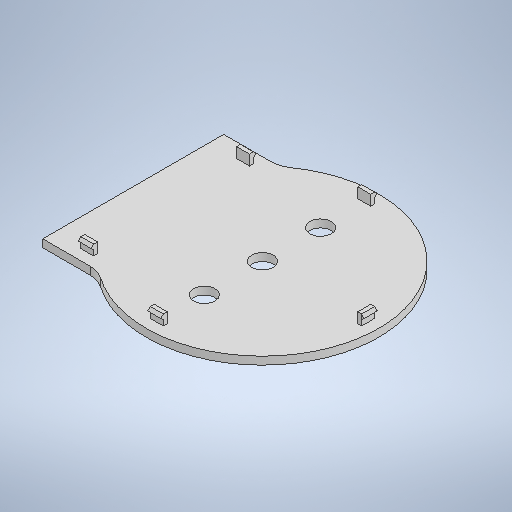
# Autodesk Inventor part: SCARA arm base - lid
Saved by Autodesk Inventor 2025.2 (Build 292293000, 293)
## iProperties
Created: 2025-01-29
Part Number: SCARA arm base - lid
Material: Generic
Document SubType Name: Modeling
Designer: caomi
Density: 1 g/cm^3
Appearance: Default
Author: caomi
Autodesk Inventor part; units mm, degrees
ref_plane "YZ Plane" through (0, 0, 0) normal (1, 0, 0) x (0, 1, 0)
ref_plane "XZ Plane" through (0, 0, 0) normal (0, 1, 0) x (-1, 0, 0)
ref_plane "XY Plane" through (0, 0, 0) normal (0, 0, 1) x (1, 0, 0)
sketch "Sketch1" plane through (0, 0, 0) normal (0, 1, 0) x (-1, 0, 0)
  circle A0 centre (0, 0) radius 45
  line L0 (28.2843, 35) -> (50, 35)
  line L1 (50, 35) -> (50, -35)
  line L2 (50, -35) -> (28.2843, -35)
  dimension "d0" = 90
  dimension "d1" = 70
  dimension "d2" = 50
  constraints: 6 end point, 2 perpendicular, 2 point on circle, 1 centre point, 1 coincident, 1 horizontal, 1 vertical alignment
  measures "d0" diameter of A0
  measures "d1" distance of L0.end L1.end
  measures "d2" distance from line of point (0, 0) L1
extrude "Extrusion1" add sketch "Sketch1" along normal blind 3
fillet "Fillet1" radius 10 2 edges at (-28.2843, 1.5, 35) (-28.2843, 1.5, -35)
sketch "Sketch3" plane through (0, 3, 0) normal (0, 1, 0) x (1, 0, 0)
  circle A0 centre (0, 0) radius 4.15
  circle A1 centre (0, -22.5) radius 4.15
  circle A2 centre (0, 22.5) radius 4.15
  line L0 (-69, 0) -> (64, 0) projected
  dimension "d16" = 45
  dimension "d17" = 8.3
  constraints: 3 centre point, 2 equal radius, 1 coincident, 1 symmetric about line, 1 vertical alignment
  measures "d16" distance of A2.centre A1.centre
  measures "d17" diameter of A0
extrude "Extrusion2" cut sketch "Sketch3" against normal blind 8.3
sketch "Sketch5" plane through (0, 3, 0) normal (0, 1, 0) x (1, 0, 0)
  arc A0 (-25.8732, -36.8182) -> (-25.8732, 36.8182) centre (0, 0) ccw projected
  arc A1 (-25.8732, -36.8182) -> (-31.6228, -35) centre (-31.6228, -45) ccw projected
  line L0 (-50, -35) -> (-31.6228, -35) projected
  line L1 (-50, 35) -> (-50, -35) projected
  line L2 (-31.6228, 35) -> (-50, 35) projected
  arc A2 (-31.6228, 35) -> (-25.8732, 36.8182) centre (-31.6228, 45) ccw projected
  arc A3 (-23.5158, -33.4636) -> (-23.5158, 33.4636) centre (0, 0) ccw
  arc A4 (-23.5158, -33.4636) -> (-31.6228, -30.9) centre (-31.6228, -45) ccw
  line L3 (-31.6228, -30.9) -> (-45.9, -30.9)
  line L4 (-45.9, -30.9) -> (-45.9, 30.9)
  line L5 (-45.9, 30.9) -> (-31.6228, 30.9)
  arc A5 (-31.6228, 30.9) -> (-23.5158, 33.4636) centre (-31.6228, 45) ccw
  arc A6 (-22.6534, -32.2364) -> (-22.6534, 32.2364) centre (0, 0) ccw
  arc A7 (-22.6534, -32.2364) -> (-31.6228, -29.4) centre (-31.6228, -45) ccw
  line L6 (-31.6228, -29.4) -> (-44.4, -29.4)
  line L7 (-44.4, -29.4) -> (-44.4, 29.4)
  line L8 (-44.4, 29.4) -> (-31.6228, 29.4)
  arc A8 (-31.6228, 29.4) -> (-22.6534, 32.2364) centre (-31.6228, 45) ccw
  line L9 (39.3206, -2.5) -> (40.8235, -2.5)
  line L10 (39.3206, 2.5) -> (40.8235, 2.5)
  line L11 (0, 0) -> (25.5499, 0) construction
  line L12 (-34.4, -30.9) -> (-34.4, -29.4)
  line L13 (-39.4, -30.9) -> (-39.4, -29.4)
  dimension "d20" = 4.1
  dimension "d21" = 1.5
  dimension "d22" = 5
  dimension "d33" = 5
  dimension "d34" = 5
  constraints: 22 end point, 16 point on circle, 6 centre point, 4 point on line, 3 horizontal, 1 perpendicular, 1 vertical, 11 other
  measures "d20" radial gap between concentric circles of A0 A3
  measures "d21" radial gap between concentric circles of A3 A6
  measures "d22" distance between parallel lines of L9 L10
  measures "d33" distance between parallel lines of L13 L12
  measures "d34" distance from line of L6.end L13
extrude "Extrusion3" add sketch "Sketch5" along normal blind 4 contours L9 A6 L10 A3
sketch "Sketch6" plane through (40.8235, 3, -2.5) normal (0, 0, -1) x (-1, 0, 0)
  line L0 (0, 4) -> (-1, 3)
  line L1 (-1, 3) -> (0, 2)
  line L2 (-1, 3) -> (-1.2746, 3) construction
  line L3 (0, 0) -> (0, 4) projected
  line L4 (0, 4) -> (0, 2)
  point P0 (40.8235, -3)
  dimension "d26" = 45
  dimension "d27" = 1
  constraints: 8 end point, 1 horizontal, 1 midpoint, 1 other
  measures "d26" angle of L1 L2
  measures "d27" distance from line of L3 L0.end
sketch3d "3D Sketch1"
  arc A0 (40.8235, 7, -2.5) -> (40.8235, 7, 2.5) centre (0, 7, 0) ccw
sweep "Sweep1" add profiles "Sketch6" path "3D Sketch1"
pattern_circular "Circular Pattern1" count 2 over 90 about axis through (0, 0, 0) along (0, -1, 0) of "Sweep1", "Extrusion3"
extrude "Extrusion5" add sketch "Sketch5" along normal up to surface (4 mm away) contours L3 L13 L6 L12
sketch "Sketch7" plane through (-34.4, 3, 30.9) normal (1, 0, 0) x (0, 0, -1)
  line L0 (-1, 3) -> (0.0311, 1.9689)
  line L1 (-1.364, 3) -> (-0.0782, 3) construction
  line L2 (0, 0) -> (0, 4) projected
  line L3 (-1, 3) -> (0, 4)
  point P0 (30.9, -3)
  point P1 (0, 2)
  dimension "d36" = 45
  dimension "d42" = 1
  constraints: 6 end point, 1 horizontal, 1 point on line, 1 other
  measures "d36" angle of L1 L0
  measures "d42" distance from line of L0.start L2
extrude "Extrusion4" add sketch "Sketch7" against normal up to surface (5 mm away)
mirror "Mirror1" about plane through (0, 0, 0) normal (0, 0, 1) of "Sweep1", "Extrusion3", "Circular Pattern1", "Extrusion4", "Extrusion5"
equation "\"d18\" = d17"
equation "\"d33\" = d22"
equation "\"d42\" = d27"
body "Solid1"
